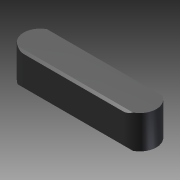
# Autodesk Inventor part: KESS5-20
Saved by Autodesk Inventor 2011 SP1 (Build 150282100, 282)
## iProperties
Created: 2016-11-23
Part Number: KESS5-20
Catalog Web Link: www.cadenas.de
Description: KED, KEDH, KEDS, KES, KESH, KESS, KEG, KEGH, KEGS-Parallel Keys
Vendor: MISUMI
Document SubType Name: Modeling
Designer: psAdmin
Manufacturer: MISUMI
Mass: 0.47024 g
Surface Area: 4.06091 cm^2
Volume: 0.47024 cm^3
Density: 1 g/cm^3
Category: PARTsolutions
Company: MISUMI
Title: KESS5-20
Author: Cadenas PARTsolutions
Comments: Parallel Keys
PSOL_IDENT_0: {$CADENAS_DATA\23d-libs\misumi\metric\28_keys_magnets\kegh.prj},214 {VTYP=3D},{NB=KESS5-20},{LINA=KE
PSOL_IDENT_1: SS5-20},{NN=KED, KEDH, KEDS, KES, KESH, KESS, KEG, KEGH, KEGS},{DATE=17.06.2016 05:51:03},{GEOMDATE=
PSOL_IDENT_2: 22.08.2013},{VERSION=},{LINEID=40},{LINESUBID=-1},{WBVAR=TYS,MAT,HARD,L,ALT1,LC}  {NB=KESS5-20},{LIN
PSOL_IDENT_3: A=KESS5-20},{KT=DUMMY},{PN=KESS5-20},{PNALG=20},{TYS=KES},{TYPEALG='KEDS','KEDS','KESS','KESS','KEGS'
PSOL_IDENT_4: ,'KEGS'},{MAT=S},{HARD=},{HARDALG='', '-'},{TS=600 or More},{B=5},{BTOL=0/-0.030},{L=20},{LALG=[10,1
PSOL_IDENT_5: 2,15,16,18,20,22,25,28,30,32,35,40,45,50,55,60]},{LALG1=[10,12,15,16,20,25,26,28,30,32,35,40,45,50]}
PSOL_IDENT_6: ,{ALT1=2},{LC=0},{LCALG=[0]},{LTOL=0/-0.21},{H=5},{HTOL=0/-0.030},{C=0.25~0.40},{C1=0.300},{CALG=[0.
PSOL_IDENT_7: 25:0.40/0.01]}
NN: KED, KEDH, KEDS, KES, KESH, KESS, KEG, KEGH, KEGS
NT: Parallel Keys
NB: KESS5-20
NBSYN: $PN.
LINA: KESS5-20
PN: KESS5-20
TYS: Round
MAT: 316 Stainless Steel
HARD: -
TS: 600 or More
B: 5
BTOL: 0/-0.030
L: 20
ALT1: w/o LC (Changes Overall Length)
LC: 0
LTOL: 0/-0.21
H: 5
HTOL: 0/-0.030
C: 0.25~0.40
SUPPLIER: MISUMI
ARTICLENO: KESS5-20
BOMINFO: KESS5-20
CREATOR: CADENAS GmbH
Autodesk Inventor part; units mm, degrees
ref_plane "YZ Plane" through (0, 0, 0) normal (1, 0, 0) x (0, 1, 0)
ref_plane "XZ Plane" through (0, 0, 0) normal (0, 1, 0) x (-1, 0, 0)
ref_plane "XY Plane" through (0, 0, 0) normal (0, 0, 1) x (1, 0, 0)
sketch "Sketch_7" plane through (0, 0, 0) normal (0, 0, 1) x (1, 0, 0)
  arc A0 (0, 2.5) -> (2.5, 0) centre (2.5, 2.5) ccw
  line L0 (2.5, 0) -> (17.5, 0)
  arc A1 (17.5, 0) -> (20, 2.5) centre (17.5, 2.5) ccw
  arc A2 (20, 2.5) -> (17.5, 5) centre (17.5, 2.5) ccw
  line L1 (17.5, 5) -> (2.5, 5)
  arc A3 (2.5, 5) -> (0, 2.5) centre (2.5, 2.5) ccw
  constraints: 8 point on circle, 4 centre point, 4 end point
extrude "Extrusion1" add sketch "Sketch_7" along normal blind 5
sketch "Sketch_8" plane through (0, 0, 0) normal (1, 0, 0) x (0, 1, 0)
  line L0 (7.5, 7.5) -> (-2.5, 7.5)
  line L1 (-2.5, 7.5) -> (-2.5, -2.5)
  line L2 (-2.5, -2.5) -> (7.5, -2.5)
  line L3 (7.5, -2.5) -> (7.5, 7.5)
  line L4 (0.3, 5) -> (0, 4.7)
  line L5 (0, 4.7) -> (0, 0.3)
  line L6 (0, 0.3) -> (0.3, 0)
  line L7 (0.3, 0) -> (4.7, 0)
  line L8 (4.7, 0) -> (5, 0.3)
  line L9 (5, 0.3) -> (5, 4.7)
  line L10 (5, 4.7) -> (4.7, 5)
  line L11 (4.7, 5) -> (0.3, 5)
  constraints: 24 end point
extrude "Extrusion2" cut sketch "Sketch_8" along normal blind 20
body "Solid1"
